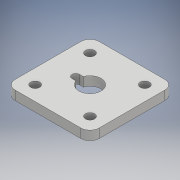
# Autodesk Inventor part: 車輪ハブ1
Saved by Autodesk Inventor 2017 (Build 210142000, 142)
## iProperties
Part Number: 車輪ハブ1
Material: 一般
Document SubType Name: Modeling
Designer: highs
Density: 1 g/cm^3
Appearance: 既定
Author: highs
Autodesk Inventor part; units mm, degrees
ref_plane "YZ Plane" through (0, 0, 0) normal (1, 0, 0) x (0, 1, 0)
ref_plane "XZ Plane" through (0, 0, 0) normal (0, 1, 0) x (-1, 0, 0)
ref_plane "XY Plane" through (0, 0, 0) normal (0, 0, 1) x (1, 0, 0)
sketch "スケッチ1" plane through (0, 0, 0) normal (0, 0, 1) x (1, 0, 0)
  line L0 (-70.6589, 70.6589) -> (71.9048, -71.9048) construction
  line L1 (17.3902, 17.3902) -> (-17.3902, -17.3902) construction
  circle A0 centre (0, 0) radius 6.05
  circle A1 centre (15, 15) radius 2.5
  circle A2 centre (-15, 15) radius 2.5
  circle A3 centre (-15, -15) radius 2.5
  circle A4 centre (15, -15) radius 2.5
  line L2 (0, 0) -> (-101.8131, 0) construction
  line L3 (-5.6921, -2.05) -> (-7.8, -2.05)
  arc A5 (-7.8, 2.05) -> (-7.8, -2.05) centre (-7.8, 0) ccw
  line L4 (-7.8, 2.05) -> (-5.6921, 2.05)
  line L5 (-7.8, -2.05) -> (-7.8, 2.05) construction
  line L6 (23, -23) -> (-23, -23)
  line L7 (-23, -23) -> (-23, 23)
  line L8 (-23, 23) -> (23, 23)
  line L9 (23, 23) -> (23, -23)
  line L10 (23, -23) -> (-23, 23) construction
  line L11 (-15, 15) -> (15, 15) construction
  line L12 (15, 15) -> (15, -15) construction
  line L13 (15, -15) -> (-15, -15) construction
  line L14 (-15, -15) -> (-15, 15) construction
  point P0 (0, 0)
  point P1 (-6.05, 0)
  dimension "d5" = 12.1
  dimension "d8" = 5
  dimension "d12" = 360
  dimension "d17" = 45
  dimension "d18" = 4.1
  dimension "d23" = 46
  dimension "d25" = 30
  dimension "d26" = 46
  dimension "d28" = 7.8
  constraints: 30 end point, 7 point on line, 6 centre point, 5 point on circle, 4 horizontal, 4 midpoint, 4 perpendicular, 2 parallel, 1 coincident, 1 vertical, 10 other
  measures "d5" diameter of A0
  measures "d8" diameter of A1
  measures "d17" angle of L0 L2
  measures "d18" distance between parallel lines of L4 L3
  measures "d23" distance of L8.end L6.start
  measures "d25" distance of L11.start L11.end
  measures "d26" distance of L7.end L8.end
  measures "d28" distance from line of L5 point (0, 0)
extrude "押し出し2" add sketch "スケッチ1" along normal blind 5
fillet "フィレット2" radius 5 4 edges at (-23, 23, 2.5) (23, 23, 2.5) (23, -23, 2.5) (-23, -23, 2.5)
